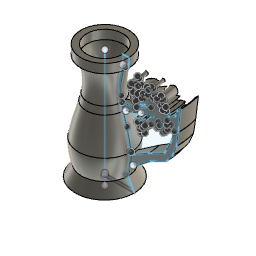
Vase v2 (Autodesk Fusion 360 design; units mm, degrees)
Autodesk Fusion 360 part; units mm, degrees
note: some values were not read from the file. Set by a fixed rule: which sketch regions a step uses.
sketch "Sketch9" plane through (0, 0, 0) normal (0, 1, 0) x (1, 0, 0)
sketch "Sketch10" plane through (0, 0, 0) normal (0, 1, 0) x (1, 0, 0)
  line L0 (0, 0) -> (14.7524, 0)
  line L1 (14.7524, 0) -> (11.6811, -5.9203)
  line L2 (0, 0) -> (0, -1.1379)
  spline S0 degree 5 poles (28.2382, -44.9084) (28.3313, -44.9262) (28.5174, -44.9618) (28.7967, -45.0152) (29.169, -45.0864) (29.6344, -45.1754) (30.0068, -45.2466) (30.286, -45.3001) (30.4722, -45.3357) (30.5653, -45.3535) knots 0 0 0 0 0 0 0.2 0.4 0.6 0.8 1 1 1 1 1 1
  spline S1 degree 5 poles (28.2382, -44.9084) (28.3276, -44.955) (28.4993, -45.0497) (28.7355, -45.1958) (29.0074, -45.3988) (29.2757, -45.6663) (29.4729, -45.9476) (29.601, -46.2422) (29.6643, -46.5497) (29.6701, -46.8688) (29.6285, -47.1977) (29.5493, -47.5326) (29.4406, -47.8671) (29.3061, -48.1914) (29.1425, -48.4911) (28.9401, -48.7477) (28.6881, -48.9429) (28.3795, -49.0613) (28.0153, -49.0944) (27.6108, -49.0442) (27.1957, -48.9239) (26.8075, -48.7532) (26.4868, -48.5551) (26.2714, -48.3521) (26.1916, -48.1626) (26.2644, -47.9974) (26.4507, -47.8889) (26.6632, -47.8215) (26.837, -47.7828) (26.932, -47.765) knots 0 0 0 0 0 0 0.04 0.08 0.12 0.16 0.2 0.24 0.28 0.32 0.36 0.4 0.44 0.48 0.52 0.56 0.6 0.64 0.68 0.72 0.76 0.8 0.84 0.88 0.92 0.96 1 1 1 1 1 1
  spline S2 degree 5 poles (26.932, -47.765) (26.9222, -47.8525) (26.9134, -48.0168) (26.9324, -48.2315) (27.0225, -48.4542) (27.2372, -48.6261) (27.5356, -48.6903) (27.8812, -48.645) (28.2109, -48.4877) (28.4496, -48.2185) (28.5298, -47.8465) (28.408, -47.393) (28.0856, -46.8985) (27.6185, -46.4233) (27.0916, -46.0331) (26.6011, -45.7871) (26.2326, -45.725) (26.0416, -45.8548) (26.0324, -46.1396) (26.1394, -46.4858) (26.2628, -46.78) (26.3011, -46.9212) (26.1856, -46.8566) (25.9114, -46.6121) (25.5171, -46.264) (25.0688, -45.9132) (24.642, -45.659) (24.3052, -45.5748) (24.1001, -45.6766) (24.0389, -45.9278) (24.1115, -46.268) (24.2898, -46.6343) (24.5336, -46.9828) (24.7949, -47.2832) (25.0231, -47.5165) (25.1697, -47.6712) (25.1934, -47.7407) (25.0643, -47.7201) (24.7613, -47.6063) (24.2713, -47.3975) (23.5867, -47.0928) (22.8808, -46.7721) (22.262, -46.4885) (21.8099, -46.2802) (21.5739, -46.1712) knots 0 0 0 0 0 0 0.025 0.05 0.075 0.1 0.125 0.15 0.175 0.2 0.225 0.25 0.275 0.3 0.325 0.35 0.375 0.4 0.425 0.45 0.475 0.5 0.525 0.55 0.575 0.6 0.625 0.65 0.675 0.7 0.725 0.75 0.775 0.8 0.825 0.85 0.875 0.9 0.925 0.95 0.975 1 1 1 1 1 1
  spline S3 degree 5 poles (21.5739, -46.1712) (21.403, -46.1905) (21.0762, -46.2208) (20.6307, -46.2417) (20.1267, -46.2199) (19.6492, -46.1089) (19.3247, -45.9144) (19.1483, -45.6405) (19.1068, -45.2965) (19.1725, -44.9007) (19.3036, -44.4809) (19.451, -44.0687) (19.565, -43.6964) (19.6011, -43.3928) (19.5271, -43.1782) (19.3277, -43.0621) (19.0634, -43.0504) (18.8065, -43.0869) (18.6092, -43.1313) (18.5041, -43.1585) knots 0 0 0 0 0 0 0.066667 0.133333 0.2 0.266667 0.333333 0.4 0.466667 0.533333 0.6 0.666667 0.733333 0.8 0.866667 0.933333 1 1 1 1 1 1
  line L3 (16.1872, -41.5362) -> (16.7391, -40.4777)
  line L4 (16.7391, -40.4777) -> (17.4139, -41.3199)
  line L5 (17.4139, -41.3199) -> (17.8704, -40.2782)
  line L6 (17.8704, -40.2782) -> (18.5452, -41.1204)
  line L7 (18.5452, -41.1204) -> (18.8784, -40.3599)
  line L8 (18.8784, -40.3599) -> (19.8103, -41.0611)
  line L9 (19.8103, -41.0611) -> (23.3214, -41.4991)
  line L10 (24.4542, -37.9884) -> (20.5941, -33.8548)
  line L11 (20.5941, -33.8548) -> (19.9909, -34.5965)
  line L12 (19.9909, -34.5965) -> (19.2789, -33.8341)
  line L13 (19.2789, -33.8341) -> (19.0445, -34.3009)
  line L14 (19.0445, -34.3009) -> (17.8373, -33.0082)
  line L15 (17.8373, -33.0082) -> (17.6436, -34.3009)
  line L16 (17.6436, -34.3009) -> (16.649, -32.5913)
  line L17 (16.649, -32.5913) -> (15.7337, -33.4461)
  line L18 (15.7337, -33.4461) -> (15.7337, -31.9571)
  line L19 (15.7337, -31.9571) -> (16.5088, -31.8571)
  spline S4 degree 5 poles (16.5088, -31.8571) (16.5346, -31.7449) (16.5852, -31.5239) (16.6583, -31.2023) (16.7501, -30.7935) (16.8564, -30.3164) (16.957, -29.8743) (17.0578, -29.4694) (17.1684, -29.1043) (17.3038, -28.7833) (17.4849, -28.5115) (17.7312, -28.2954) (18.054, -28.1428) (18.4505, -28.0622) (18.8945, -28.0639) (19.3389, -28.1575) (19.7291, -28.3487) (20.0133, -28.6361) (20.1536, -29.0078) (20.1394, -29.4367) (19.9903, -29.8815) (19.7444, -30.2932) (19.4492, -30.6214) (19.153, -30.8204) (18.8942, -30.8553) (18.6947, -30.7074) (18.591, -30.4361) (18.5461, -30.1458) (18.5307, -29.9138) (18.5266, -29.7882) knots 0 0 0 0 0 0 0.04 0.08 0.12 0.16 0.2 0.24 0.28 0.32 0.36 0.4 0.44 0.48 0.52 0.56 0.6 0.64 0.68 0.72 0.76 0.8 0.84 0.88 0.92 0.96 1 1 1 1 1 1
  spline S5 degree 5 poles (18.5266, -29.7882) (18.5413, -29.8369) (18.5733, -29.9273) (18.6295, -30.0417) (18.7211, -30.1518) (18.862, -30.2187) (19.0256, -30.2164) (19.2042, -30.1491) (19.3844, -30.0245) (19.5486, -29.8535) (19.6782, -29.6497) (19.7564, -29.4288) (19.7705, -29.2078) (19.7151, -29.0044) (19.5914, -28.8359) (19.4057, -28.7169) (19.1691, -28.6581) (18.8961, -28.6642) (18.6042, -28.733) (18.312, -28.8579) (18.0382, -29.0293) (17.8002, -29.2362) (17.613, -29.4683) (17.4871, -29.7174) (17.4291, -29.9782) (17.4423, -30.2474) (17.5108, -30.4681) (17.5948, -30.6365) (17.6652, -30.7499) (17.704, -30.807) knots 0 0 0 0 0 0 0.04 0.08 0.12 0.16 0.2 0.24 0.28 0.32 0.36 0.4 0.44 0.48 0.52 0.56 0.6 0.64 0.68 0.72 0.76 0.8 0.84 0.88 0.92 0.96 1 1 1 1 1 1
  spline S6 degree 5 poles (17.0688, -44.5361) (17.0689, -44.5353) (17.0705, -44.5358) (17.0769, -44.5425) (17.0749, -44.5342) (17.0018, -44.4334) (16.8378, -44.2539) (16.5812, -44.0399) (16.2466, -43.8524) (15.8583, -43.7403) (15.4465, -43.7298) (15.0436, -43.8305) (14.6812, -44.0385) (14.3864, -44.3398) (14.1791, -44.7145) (14.0675, -45.1399) (14.0481, -45.5935) (14.1098, -46.0538) (14.2368, -46.5018) (14.4116, -46.9222) (14.6184, -47.305) (14.8459, -47.6463) (15.0912, -47.9503) (15.3578, -48.2276) (15.6508, -48.4921) (15.9738, -48.7586) (16.3248, -49.04) (16.6922, -49.3446) (17.0512, -49.6734) (17.3606, -50.0182) (17.5755, -50.3643) (17.6571, -50.6942) (17.5851, -50.9902) (17.3665, -51.2377) (17.0513, -51.4282) (16.7268, -51.5605) (16.4857, -51.6363) (16.4015, -51.6582) (16.4999, -51.6259) (16.7336, -51.5339) (17.0147, -51.3758) (17.2441, -51.1475) (17.3432, -50.8523) (17.2834, -50.504) (17.0744, -50.1235) (16.7521, -49.7354) (16.367, -49.3645) (15.9719, -49.0319) (15.6113, -48.7518) (15.3068, -48.5271) (15.0562, -48.3498) (14.8431, -48.2049) (14.6446, -48.0745) (14.4385, -47.9405) (14.2126, -47.7889) (13.9679, -47.6117) (13.7133, -47.4055) (13.4631, -47.1707) (13.2328, -46.9109) (13.0357, -46.6318) (12.8802, -46.3406) (12.7713, -46.0452) (12.7105, -45.7532) (12.6974, -45.4715) (12.7297, -45.2049) (12.804, -44.9558) (12.9166, -44.7252) (13.0635, -44.5128) (13.2415, -44.3178) (13.4482, -44.1396) (13.6822, -43.9778) (13.8906, -43.8614) (14.0587, -43.7814) (14.1761, -43.7313) (14.2361, -43.707) knots 0 0 0 0 0 0 0.01428571 0.02857143 0.04285714 0.05714286 0.07142857 0.08571429 0.1 0.11428571 0.12857143 0.14285714 0.15714286 0.17142857 0.18571429 0.2 0.21428571 0.22857143 0.24285714 0.25714286 0.27142857 0.28571429 0.3 0.31428571 0.32857143 0.34285714 0.35714286 0.37142857 0.38571429 0.4 0.41428571 0.42857143 0.44285714 0.45714286 0.47142857 0.48571429 0.5 0.51428571 0.52857143 0.54285714 0.55714286 0.57142857 0.58571429 0.6 0.61428571 0.62857143 0.64285714 0.65714286 0.67142857 0.68571429 0.7 0.71428571 0.72857143 0.74285714 0.75714286 0.77142857 0.78571429 0.8 0.81428571 0.82857143 0.84285714 0.85714286 0.87142857 0.88571429 0.9 0.91428571 0.92857143 0.94285714 0.95714286 0.97142857 0.98571429 1 1 1 1 1 1
  line L20 (16.9037, -45.6738) -> (17.234, -43.3983)
  spline S7 degree 5 poles (18.5041, -43.1585) (18.4847, -43.1957) (18.4455, -43.269) (18.3856, -43.3763) (18.3034, -43.5134) (18.1947, -43.6702) (18.1002, -43.7765) (18.0229, -43.8401) (17.968, -43.8741) (17.9397, -43.8891) knots 0 0 0 0 0 0 0.2 0.4 0.6 0.8 1 1 1 1 1 1
  line L21 (18.0148, -43.8494) -> (17.8647, -43.9287)
  line L22 (17.9397, -43.8891) -> (17.9538, -44.0124)
  spline S8 degree 5 poles (17.9538, -44.0124) (17.9004, -44.1103) (17.7976, -44.3028) (17.6551, -44.582) (17.4887, -44.9351) (17.32, -45.3446) (17.1908, -45.7233) (17.101, -46.0726) (17.0511, -46.3954) (17.0413, -46.6959) (17.072, -46.9801) (17.1435, -47.2546) (17.2564, -47.5239) (17.4112, -47.7893) (17.6086, -48.0458) (17.8489, -48.282) (18.1323, -48.4836) (18.4582, -48.6368) (18.8249, -48.7318) (19.2289, -48.7661) (19.6655, -48.7475) (20.1281, -48.6907) (20.6091, -48.6152) (21.1, -48.5419) (21.5916, -48.491) (22.0745, -48.4791) (22.539, -48.5163) (22.9755, -48.6046) (23.3746, -48.7409) (23.7264, -48.9178) (24.0209, -49.1262) (24.2477, -49.3564) (24.3958, -49.6009) (24.4545, -49.8539) (24.4181, -50.1071) (24.289, -50.3468) (24.0825, -50.5487) (23.8275, -50.6799) (23.5626, -50.7134) (23.3312, -50.6382) (23.1798, -50.476) (23.1487, -50.279) (23.2547, -50.1) (23.4716, -49.9644) (23.7242, -49.8546) (23.924, -49.7382) (23.9934, -49.5847) (23.9018, -49.3922) (23.6683, -49.1891) (23.3372, -49.0144) (22.962, -48.9061) (22.5837, -48.8833) (22.2194, -48.9386) (21.8708, -49.048) (21.5287, -49.1781) (21.1797, -49.294) (20.8112, -49.3668) (20.4178, -49.3819) (20.0009, -49.3377) (19.5671, -49.2409) (19.1262, -49.1033) (18.6902, -48.9381) (18.2713, -48.7564) (17.881, -48.5632) (17.5282, -48.3566) (17.2205, -48.1316) (16.963, -47.8816) (16.7586, -47.6014) (16.608, -47.2891) (16.5092, -46.9493) (16.4584, -46.5916) (16.4504, -46.2283) (16.4799, -45.8728) (16.542, -45.5373) (16.6329, -45.231) (16.7506, -44.959) (16.8653, -44.7709) (16.9626, -44.6469) (17.0326, -44.5717) (17.0688, -44.5361) knots 0 0 0 0 0 0 0.01333333 0.02666667 0.04 0.05333333 0.06666667 0.08 0.09333333 0.10666667 0.12 0.13333333 0.14666667 0.16 0.17333333 0.18666667 0.2 0.21333333 0.22666667 0.24 0.25333333 0.26666667 0.28 0.29333333 0.30666667 0.32 0.33333333 0.34666667 0.36 0.37333333 0.38666667 0.4 0.41333333 0.42666667 0.44 0.45333333 0.46666667 0.48 0.49333333 0.50666667 0.52 0.53333333 0.54666667 0.56 0.57333333 0.58666667 0.6 0.61333333 0.62666667 0.64 0.65333333 0.66666667 0.68 0.69333333 0.70666667 0.72 0.73333333 0.74666667 0.76 0.77333333 0.78666667 0.8 0.81333333 0.82666667 0.84 0.85333333 0.86666667 0.88 0.89333333 0.90666667 0.92 0.93333333 0.94666667 0.96 0.97333333 0.98666667 1 1 1 1 1 1
  line L23 (15.5154, -40.03) -> (15.7145, -40.4529)
  line L24 (15.5154, -40.03) -> (15.5171, -40.3233)
  spline S9 degree 5 poles (14.2361, -43.707) (14.2054, -43.597) (14.1479, -43.3833) (14.0733, -43.0814) (13.9973, -42.7164) (13.9415, -42.3232) (13.925, -41.9938) (13.9474, -41.7287) (14.0077, -41.5282) (14.1037, -41.3919) (14.2322, -41.3185) (14.388, -41.3056) (14.5646, -41.3482) (14.7538, -41.4366) (14.9463, -41.5544) (15.1314, -41.6768) (15.2971, -41.7683) (15.4324, -41.7918) (15.5289, -41.7188) (15.5831, -41.5384) (15.5989, -41.2702) (15.5868, -40.9605) (15.5603, -40.665) (15.533, -40.4363) (15.5151, -40.308) (15.5111, -40.2826) (15.5145, -40.3062) (15.5166, -40.3202) (15.5171, -40.3233) (15.5171, -40.3233) knots 0 0 0 0 0 0 0.04 0.08 0.12 0.16 0.2 0.24 0.28 0.32 0.36 0.4 0.44 0.48 0.52 0.56 0.6 0.64 0.68 0.72 0.76 0.8 0.84 0.88 0.92 0.96 1 1 1 1 1 1
  line L25 (15.5163, -40.8377) -> (15.5178, -39.8089)
  spline S10 degree 5 poles (15.7145, -40.4529) (15.7276, -40.4784) (15.7553, -40.5347) (15.8021, -40.6346) (15.8734, -40.7947) (15.9723, -41.0247) (16.0563, -41.2233) (16.1211, -41.3777) (16.165, -41.483) (16.1872, -41.5362) knots 0 0 0 0 0 0 0.2 0.4 0.6 0.8 1 1 1 1 1 1
  line L26 (15.6812, -40.3876) -> (15.7479, -40.5182)
  line L27 (30.73, -43.6304) -> (32.6992, -43.713)
  line L28 (32.6992, -43.713) -> (32.0394, -41.8578)
  spline S11 degree 5 poles (31.1379, -37.9052) (31.1318, -37.9949) (31.1214, -38.1736) (31.1114, -38.4396) (31.1098, -38.79) (31.1369, -39.2173) (31.1966, -39.5451) (31.2736, -39.7791) (31.3414, -39.9291) (31.3795, -40.0025) knots 0 0 0 0 0 0 0.2 0.4 0.6 0.8 1 1 1 1 1 1
  line L29 (31.3461, -39.938) -> (31.413, -40.067)
  spline S12 degree 5 poles (30.73, -43.6304) (30.6127, -43.5771) (30.3884, -43.4785) (30.0829, -43.3543) (29.7383, -43.2371) (29.419, -43.1764) (29.22, -43.2081) (29.149, -43.3384) (29.2068, -43.5679) (29.3851, -43.8901) (29.6731, -44.2969) (29.9836, -44.6838) (30.2583, -45.0063) (30.4599, -45.2354) (30.5653, -45.3535) knots 0 0 0 0 0 0 0.1 0.2 0.3 0.4 0.5 0.6 0.7 0.8 0.9 1 1 1 1 1 1
  line L30 (20.1857, -32.9632) -> (20.1857, -32.0056)
  spline S13 degree 5 poles (17.704, -30.807) (17.7284, -30.8575) (17.7786, -30.9578) (17.8583, -31.1063) (17.9732, -31.3) (18.1315, -31.5349) (18.3043, -31.7622) (18.4909, -31.981) (18.6897, -32.1904) (18.8972, -32.3892) (19.1087, -32.5759) (19.3181, -32.7476) (19.5189, -32.8993) (19.7048, -33.0236) (19.8697, -33.1094) (20.0086, -33.1414) (20.0958, -33.1115) (20.1466, -33.0523) (20.1738, -32.9958) (20.1857, -32.9632) knots 0 0 0 0 0 0 0.066667 0.133333 0.2 0.266667 0.333333 0.4 0.466667 0.533333 0.6 0.666667 0.733333 0.8 0.866667 0.933333 1 1 1 1 1 1
  line L31 (20.0418, -33.3555) -> (20.3297, -32.571)
  spline S14 degree 5 poles (20.1857, -32.0663) (20.2031, -32.111) (20.2354, -32.2006) (20.277, -32.3357) (20.3444, -32.5219) (20.5624, -32.7842) (20.9773, -33.0841) (21.5593, -33.4103) (22.2343, -33.7401) (22.9132, -34.044) (23.526, -34.2916) (24.0612, -34.4568) (24.5776, -34.523) (25.1581, -34.4842) (25.875, -34.3485) (26.7544, -34.139) (27.7311, -33.8984) (28.637, -33.6865) (29.2746, -33.5638) (29.4804, -33.5766) (29.1826, -33.7432) (28.4841, -34.0349) (27.6439, -34.3809) (26.9685, -34.6967) (26.7262, -34.907) (27.0574, -34.9683) (27.8712, -34.8963) (28.9154, -34.7492) (29.8709, -34.6046) (30.4416, -34.5382) (30.4354, -34.604) (29.8763, -34.8079) (28.9835, -35.1104) (28.066, -35.4495) (27.4383, -35.7574) (27.3363, -35.9784) (27.8112, -36.0907) (28.7293, -36.1075) (29.8529, -36.063) (30.8975, -36.0028) (31.5983, -35.9727) (31.7718, -36.008) (31.3839, -36.1219) (30.5185, -36.3102) (29.3421, -36.556) (28.0697, -36.8345) (26.9299, -37.1182) (26.1317, -37.381) (25.8266, -37.6041) (26.1133, -37.7753) (27.0501, -37.8871) (28.342, -37.9263) (29.6199, -37.927) (30.609, -37.9146) (31.1379, -37.9052) knots 0 0 0 0 0 0 0.02 0.04 0.06 0.08 0.1 0.12 0.14 0.16 0.18 0.2 0.22 0.24 0.26 0.28 0.3 0.32 0.34 0.36 0.38 0.4 0.42 0.44 0.46 0.48 0.5 0.52 0.54 0.56 0.58 0.6 0.62 0.64 0.66 0.68 0.7 0.72 0.74 0.76 0.78 0.8 0.82 0.84 0.86 0.88 0.9 0.92 0.94 0.96 0.98 1 1 1 1 1 1
  line L32 (19.6638, -30.7212) -> (20.7076, -33.4114)
  spline S15 degree 5 poles (35, -37) (34.9439, -37.1348) (34.83, -37.3943) (34.6535, -37.7531) (34.407, -38.1697) (34.0789, -38.5803) (33.729, -38.8708) (33.3554, -39.031) (32.9571, -39.055) (32.535, -38.9475) (32.0907, -38.7183) (31.7191, -38.4453) (31.4318, -38.1933) (31.2365, -38.0047) (31.1379, -37.9052) knots 0 0 0 0 0 0 0.1 0.2 0.3 0.4 0.5 0.6 0.7 0.8 0.9 1 1 1 1 1 1
  line L33 (0, 4) -> (0, -55)
  spline S16 degree 2 poles (13.8858, -34.6304) (18.1752, -36.5668) (24.4542, -37.9884) knots 0 0 0 1.11198 1.11198 1.11198 weights 1 3 1
  line L34 (32.0394, -41.8578) -> (35.4076, -43.6238)
  line L35 (35.4076, -43.6238) -> (36.4145, -46.4548)
  line L36 (36.4145, -46.4548) -> (38.0001, -48)
  line L37 (36.872, -37.4341) -> (38.0001, -48)
  spline S17 degree 2 poles (11.6811, -5.9203) (14.2272, -11.887) (13.2168, -17.1379) knots 0 0 0 1.137519 1.137519 1.137519 weights 1 0.470351 1
  spline S18 degree 5 poles (13.2168, -17.1379) (13.1604, -17.5394) (13.0387, -18.3479) (12.8294, -19.5774) (12.4967, -21.2502) (11.992, -23.3982) (11.4054, -25.6041) (10.7536, -27.8678) (10.0694, -30.1864) (9.4019, -32.5547) (8.8079, -34.9658) (8.3453, -37.4123) (8.0656, -39.8874) (8.0049, -42.3853) (8.1801, -44.9018) (8.5961, -47.4344) (9.1198, -49.4719) (9.6182, -51.0062) (9.997, -52.0317) (10.1981, -52.5452) knots 0 0 0 0 0 0 0.066667 0.133333 0.2 0.266667 0.333333 0.4 0.466667 0.533333 0.6 0.666667 0.733333 0.8 0.866667 0.933333 1 1 1 1 1 1
  line L38 (0, -1.2626) -> (12.675, -1.2626)
  line L39 (12.675, -1.2626) -> (10.286, -5.8678)
  spline S19 degree 3 poles (10.286, -5.8678) (10.3639, -6.0505) (10.4419, -6.2331) (10.5198, -6.4158) (10.7134, -6.8693) (11.0053, -7.7758) (11.2835, -9.0558) (11.602, -10.5208) (11.8844, -12.4509) (11.9967, -13.9677) (12.1014, -15.3818) (12.0589, -16.3932) (11.9915, -16.816) (11.9866, -16.8467) (11.9817, -16.8745) (11.9769, -16.8993) (11.9749, -16.9097) (11.9729, -16.9202) (11.9709, -16.9306) knots -0.111067 -0.111067 -0.111067 -0.111067 0 0 0 0.345852 0.345852 0.345852 0.741686 0.741686 0.741686 1.110697 1.110697 1.110697 1.137519 1.137519 1.137519 1.144739 1.144739 1.144739 1.144739
  spline S20 degree 3 poles (11.9709, -16.9306) (11.9694, -16.9411) (11.9679, -16.9517) (11.9664, -16.9622) (11.5845, -19.6814) (10.9326, -22.564) (10.0698, -25.651) (9.0858, -29.1718) (7.8016, -32.9882) (7.1741, -37.0234) (6.6698, -40.2664) (6.6542, -43.6305) (7.2818, -47.0006) (7.6537, -48.9982) (8.2373, -51.0004) (9.0224, -53.0055) knots -0.00105 -0.00105 -0.00105 -0.00105 0 0 0 0.277751 0.277751 0.277751 0.594523 0.594523 0.594523 0.849105 0.849105 0.849105 1 1 1 1
  line L40 (10.1981, -52.5452) -> (10.3929, -53.0427)
  spline S21 degree 2 poles (9.2874, -33.0805) (10.5657, -33.7651) (13.8858, -34.6304) knots 0 0 0 0.486734 0.486734 0.486734 weights 1 3 1
  spline S22 degree 5 poles (8.5398, -36.5061) (8.8487, -36.5322) (9.4652, -36.5909) (10.3866, -36.6985) (11.6081, -36.8815) (13.1222, -37.1805) (14.6226, -37.5559) (16.1082, -38.0139) (17.5785, -38.5571) (19.0341, -39.1818) (20.4763, -39.8817) (21.6201, -40.4966) (22.4727, -40.9868) (23.0389, -41.3262) (23.3214, -41.4991) knots 0 0 0 0 0 0 0.1 0.2 0.3 0.4 0.5 0.6 0.7 0.8 0.9 1 1 1 1 1 1
  line L41 (12.7771, -10.1088) -> (23, -18)
  line L42 (23, -18) -> (31, -22)
  line L43 (31, -22) -> (34, -26)
  line L44 (34, -26) -> (36, -31)
  line L45 (36, -31) -> (36.872, -37.4341)
  line L46 (13.3213, -15.9763) -> (22, -21)
  line L47 (22, -21) -> (30, -25)
  line L48 (30, -25) -> (33, -31)
  line L49 (33, -31) -> (35, -37)
  line L50 (12, -53.0055) -> (12, -57.5088)
  line L51 (12, -57.5088) -> (9.0224, -57.5088)
  line L52 (9.0224, -57.5088) -> (9.0224, -53.0055)
  line L53 (10.3929, -53.0427) -> (12, -53.0055)
  point P0 (18.6043, -32.0978)
  point P1 (19.6876, -33.0068)
  point P2 (20.5022, -32.6884)
  point P3 (23.305, -34.196)
  point P4 (26.5292, -34.1907)
  point P5 (29.2822, -33.6731)
  point P6 (26.8789, -34.8872)
  point P7 (30.3656, -34.5821)
  point P8 (27.4641, -35.8398)
  point P9 (31.4925, -35.9893)
  point P10 (26.8613, -37.1577)
  point P11 (29.1919, -43.3048)
  point P12 (29.6253, -46.3991)
  point P13 (29.356, -48.0597)
  point P14 (28.1773, -49.0686)
  point P15 (26.3038, -48.3535)
  point P16 (27.5981, -48.663)
  point P17 (28.4092, -47.5045)
  point P18 (26.0923, -45.8822)
  point P19 (26.266, -46.867)
  point P20 (24.5283, -45.6503)
  point P21 (24.1227, -46.2295)
  point P22 (25.1256, -47.6325)
  point P23 (19.1373, -45.4132)
  point P24 (19.5757, -43.4773)
  point P25 (17.0697, -44.5303)
  point P26 (16.3824, -43.9402)
  point P27 (14.2961, -44.5315)
  point P28 (14.6802, -47.3868)
  point P29 (16.647, -49.3131)
  point P30 (17.4493, -51.1204)
  point P31 (16.4464, -51.6448)
  point P32 (17.2099, -51.1341)
  point P33 (15.8072, -48.9064)
  point P34 (14.5227, -47.9949)
  point P35 (13.3065, -46.9861)
  point P36 (12.7078, -45.527)
  point P37 (13.1056, -44.4753)
  point P38 (14.1307, -41.3911)
  point P39 (14.9529, -41.5608)
  point P40 (15.5477, -41.6266)
  point P41 (15.5171, -40.3233)
  point P42 (17.1629, -29.1482)
  point P43 (18.2557, -28.113)
  point P44 (20.077, -28.8651)
  point P45 (19.2158, -30.7544)
  point P46 (19.0681, -30.1908)
  point P47 (19.7439, -29.4108)
  point P48 (19.237, -28.6855)
  point P49 (17.7151, -29.353)
  point P50 (17.0554, -46.4602)
  point P51 (17.3775, -47.719)
  point P52 (18.7817, -48.7072)
  point P53 (21.9075, -48.4896)
  point P54 (24.1513, -49.2708)
  point P55 (24.3249, -50.2556)
  point P56 (23.4269, -50.6541)
  point P57 (23.2412, -50.1572)
  point P58 (23.9385, -49.6615)
  point P59 (23.0796, -48.952)
  point P60 (21.11, -49.2993)
  point P61 (18.5066, -48.8554)
  point P62 (16.7367, -47.5319)
  point P63 (16.5138, -45.7134)
  point P64 (33.3281, -39.0019)
  point P65 (8.178, -39.1712)
  point P66 (11, -27)
  point P67 (16, -38)
  dimension "d15" = 1.2626
  constraint coincident L0.start L2.start
  constraint horizontal L0
  constraint coincident S7.end L22.start
  constraint parallel L4 L6
  constraint parallel L5 L7
  constraint parallel L10 L12
  constraint parallel L12 L14
  constraint perpendicular L14 L17
  constraint midpoint S6.start L20
  constraint midpoint S7.end L21
  constraint coincident L23.end S10
  constraint coincident P41 L24.end
  constraint coincident L24 P41
  constraint midpoint P41 L25
  constraint coincident L23 S10.start
  constraint midpoint L23.end L26
  constraint coincident L27.start S12.start
  constraint midpoint S11.end L29
  constraint coincident L30.start S13.end
  constraint midpoint L30.start L31
  constraint coincident L30 S14.start
  constraint midpoint S14.start L32
  constraint perpendicular L0 L33
  constraint parallel L28 L35
  constraint coincident S18 S21.start
  constraint coincident S18 S22.start
  constraint coincident S17 L41.start
  constraint coincident S17 L46.start
  constraint vertical L50
  constraint horizontal L51
  constraint vertical L52
revolve "Revolve6" add sketch "Sketch10" angle 16 about axis through (0, 0, -4) along (0, 0, 1) contours S0 S1 S2 S3 L3 L4 L5 L6 L7 L8 L9 L10 L11 L12 L13 L14 L15 L16 L17 L18 L19 S4 S5 S6 S7 L22 S8 L23 S9 L25 S10 L26 L27 L28 S12 L30 S13 S14 S15 S16 L34 L35 L36 L37 S17 S18 S21 S22 L41 L42 L43 L44 L45 L46 L47 L48 L49 | L23 L24 L25 picked at (26.3312, -40.8552) picked at (15.5166, -40.1292) makes body 1
revolve "Revolve1" add sketch "Sketch10" angle 360 about axis through (0, 0, -4) along (0, 0, 1) separate body contours L0 L1 L2 L33 S17 S18 L38 L39 S19 S20 L40 L50 L51 L52 L53 picked at (10.4718, -56.0201) makes body 2
named bodies: "Vase", "Handle"
